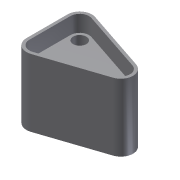
# Autodesk Inventor part: JointC4_
Saved by Autodesk Inventor 2011 SP1 (Build 150282100, 282)
## iProperties
Created: 2012-12-12
Part Number: JointC4_
Document SubType Name: Modeling
Designer: arihon
Density: 1 g/cm^3
Author: arihon
Autodesk Inventor part; units mm, degrees
ref_plane "YZ Plane" through (0, 0, 0) normal (1, 0, 0) x (0, 1, 0)
ref_plane "XZ Plane" through (0, 0, 0) normal (0, 1, 0) x (-1, 0, 0)
ref_plane "XY Plane" through (0, 0, 0) normal (0, 0, 1) x (1, 0, 0)
sketch "スケッチ1" plane through (0, 0, 0) normal (0, 0, 1) x (1, 0, 0)
  arc A0 (-3.6033, 4.0671) -> (-5.469, 7.7986) centre (-6.4019, 5) ccw
  arc A1 (-9.3519, -5) -> (-5.469, -7.7986) centre (-6.4019, -5) ccw
  arc A2 (5.7995, 0.9329) -> (9.531, -2.7986) centre (8.5981, 0) ccw
  line L0 (-9.3519, 5) -> (-9.3519, -5)
  line L1 (8.5981, 0) -> (-6.4019, 5)
  line L2 (-6.4019, 5) -> (-5.469, 7.7986)
  line L3 (-5.469, 7.7986) -> (9.531, 2.7986)
  line L4 (8.5981, 0) -> (-6.4019, -5)
  line L5 (-6.4019, -5) -> (-5.469, -7.7986)
  line L6 (-5.469, -7.7986) -> (9.531, -2.7986)
  arc A3 (-9.3519, 5) -> (-3.6033, 4.0671) centre (-6.4019, 5) ccw
  arc A4 (-3.6033, -4.0671) -> (-9.3519, -5) centre (-6.4019, -5) ccw
  arc A5 (-5.469, -7.7986) -> (-3.6033, -4.0671) centre (-6.4019, -5) ccw
  arc A6 (-5.469, 7.7986) -> (-9.3519, 5) centre (-6.4019, 5) ccw
  arc A7 (9.531, 2.7986) -> (5.7995, 0.9329) centre (8.5981, 0) ccw
  arc A8 (9.531, -2.7986) -> (9.531, 2.7986) centre (8.5981, 0) ccw
  point P0 (0, 0)
  dimension "d0" = 15
  dimension "d1" = 15
  dimension "d2" = 10
  dimension "d3" = 5
  dimension "d4" = 0
  dimension "d5" = 5.9
  dimension "d6" = 5.9
  dimension "d7" = 5.9
  constraints: 18 point on circle, 14 end point, 9 centre point, 6 tangent, 3 coincident, 3 point on line, 2 perpendicular
  measures "d0" horizontal distance of point (-6.402, 5) point (8.598, 0)
  measures "d1" horizontal distance of point (8.598, 0) point (-6.402, -5)
  measures "d2" distance of point (-6.402, -5) point (-6.402, 5)
  measures "d3" vertical distance of point (-6.402, -5) point (8.598, 0)
  measures "d4" vertical distance of point (8.598, 0) point (0, 0)
  measures "d5" diameter of A0
  measures "d6" diameter of A1
  measures "d7" diameter of A2
extrude "押し出し1" add sketch "スケッチ1" along normal blind 16.4
sketch "スケッチ2" plane through (0, 0, 16.4) normal (0, 0, 1) x (1, 0, 0)
  arc A0 (9.531, -2.7986) -> (9.531, 2.7986) centre (8.5981, 0) ccw projected
  arc A1 (-5.469, 7.7986) -> (-9.3519, 5) centre (-6.4019, 5) ccw projected
  arc A2 (-9.3519, -5) -> (-5.469, -7.7986) centre (-6.4019, -5) ccw projected
  point P0 (0, 0)
  constraints: 3 coincident
hole "Hole1" at (-6.4019, 5, 16.4) at (-6.4019, -5, 16.4) at (8.5981, 0, 16.4) direction (0, 0, -1) diameter 3.2 depth 8
sketch "スケッチ3" plane through (0, 0, 16.4) normal (0, 0, 1) x (1, 0, 0)
  circle A0 centre (8.5981, 0) radius 1.6 projected
  circle A1 centre (-6.4019, -5) radius 1.6 projected
  line L0 (9.531, -2.7986) -> (-5.469, -7.7986) projected
  arc A2 (9.531, -2.7986) -> (9.531, 2.7986) centre (8.5981, 0) ccw projected
  line L1 (-5.469, 7.7986) -> (9.531, 2.7986) projected
  arc A3 (-5.469, 7.7986) -> (-9.3519, 5) centre (-6.4019, 5) ccw projected
  arc A4 (-9.3519, -5) -> (-5.469, -7.7986) centre (-6.4019, -5) ccw projected
  arc A5 (-8.6519, 5) -> (-5.6904, 7.1345) centre (-6.4019, 5) ccw
  arc A6 (-5.6904, -7.1345) -> (-8.6519, -5) centre (-6.4019, -5) ccw
  arc A7 (9.3096, 2.1345) -> (9.3096, -2.1345) centre (8.5981, 0) ccw
  line L2 (-8.6519, 5) -> (-8.6519, -5)
  circle A8 centre (-6.4019, -5) radius 1.6 projected
  line L3 (-6.4019, -5) -> (8.5981, 0)
  line L4 (8.5981, 0) -> (9.3096, -2.1345)
  line L5 (-5.6904, -7.1345) -> (9.3096, -2.1345)
  line L6 (8.5981, 0) -> (-6.4019, 5)
  line L7 (-6.4019, 5) -> (-5.6904, 7.1345)
  line L8 (-5.6904, 7.1345) -> (9.3096, 2.1345)
  arc A9 (-5.6904, 7.1345) -> (-8.6519, 5) centre (-6.4019, 5) ccw
  arc A10 (-8.6519, -5) -> (-5.6904, -7.1345) centre (-6.4019, -5) ccw
  arc A11 (9.3096, -2.1345) -> (9.3096, 2.1345) centre (8.5981, 0) ccw
  point P0 (0, 0)
  dimension "d17" = 4.5
  dimension "d18" = 4.5
  dimension "d19" = 4.5
  constraints: 14 end point, 12 point on circle, 6 centre point, 3 coincident, 3 tangent, 2 parallel, 2 perpendicular
  measures "d17" diameter of A5
  measures "d18" diameter of A6
  measures "d19" diameter of A7
extrude "押し出し2" cut sketch "スケッチ3" against normal blind 4 contours A0 L6 A7 A11 L4 | A0 L3 A7 L6 | L4 A7 L3 A0 | L6 A5 L8 A7 | A7 L3 A6 L2 A5 L6 | L5 A6 L3 A7 | L6 L7 A5 | A5 A9 L7 L6 | A10 A6
equation "\"d1\" = d0"
equation "\"d3\" = 0.5 * d2"
